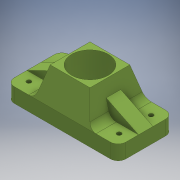
# Autodesk Inventor part: sujetador guia ejercedor presion
Saved by Autodesk Inventor 2018 (Build 220112000, 112)
## iProperties
Created: 2019-05-18
Part Number: sujetador guia ejercedor presion
Material: Generic
Document SubType Name: Modeling
Designer: JLVega003
Density: 1 g/cm^3
Appearance: Olive Green
Author: JLVega003
Autodesk Inventor part; units mm, degrees
ref_plane "YZ Plane" through (0, 0, 0) normal (1, 0, 0) x (0, 1, 0)
ref_plane "XZ Plane" through (0, 0, 0) normal (0, 1, 0) x (-1, 0, 0)
sketch "Sketch1" plane through (0, 0, 0) normal (0, 0, 1) x (1, 0, 0)
  line L0 (57.5, -28.5) -> (-57.5, -28.5)
  line L1 (-57.5, -28.5) -> (-57.5, 28.5)
  line L2 (-57.5, 28.5) -> (57.5, 28.5)
  line L3 (57.5, 28.5) -> (57.5, -28.5)
  line L4 (57.5, -28.5) -> (-57.5, 28.5) construction
  line L5 (-57.5, -28.5) -> (57.5, 28.5) construction
  line L6 (46.5, -16.5) -> (-46.5, -16.5) construction
  line L7 (-46.5, -16.5) -> (-46.5, 16.5) construction
  line L8 (-46.5, 16.5) -> (46.5, 16.5) construction
  line L9 (46.5, 16.5) -> (46.5, -16.5) construction
  line L10 (46.5, -16.5) -> (-46.5, 16.5) construction
  line L11 (-46.5, -16.5) -> (46.5, 16.5) construction
  line L12 (36, -11.5) -> (-36, -11.5) construction
  line L13 (-36, -11.5) -> (-36, 11.5) construction
  line L14 (-36, 11.5) -> (36, 11.5) construction
  line L15 (36, 11.5) -> (36, -11.5) construction
  line L16 (36, -11.5) -> (-36, 11.5) construction
  line L17 (-36, -11.5) -> (36, 11.5) construction
  circle A0 centre (-46.5, 16.5) radius 2.25
  circle A1 centre (-46.5, -16.5) radius 2.25
  circle A2 centre (46.5, -16.5) radius 2.25
  circle A3 centre (46.5, 16.5) radius 2.25
  point P0 (0, 0)
  dimension "d0" = 115
  dimension "d1" = 57
  dimension "d2" = 93
  dimension "d3" = 33
  dimension "d4" = 72
  dimension "d5" = 23
  dimension "d6" = 4.5
  constraints: 36 end point, 6 midpoint, 6 parallel, 4 centre point, 4 coincident, 3 equal radius, 3 horizontal, 3 perpendicular
  measures "d0" distance of L1.end L2.end
  measures "d1" distance of L0.end L1.end
  measures "d2" distance of L7.end L8.end
  measures "d3" distance of L6.end L7.end
  measures "d4" distance of L13.end L14.end
  measures "d5" distance of L12.end L13.end
  measures "d6" diameter of A0
extrude "Extrusion1" add sketch "Sketch1" along normal blind 15
sketch "Sketch6" plane through (0, 0, 15) normal (0, 0, 1) x (1, 0, 0)
  line L0 (57.5, 28.5) -> (-57.5, 28.5) projected
  line L1 (28.5, -28.5) -> (-28.5, -28.5)
  line L2 (-28.5, -28.5) -> (-28.5, 28.5)
  line L3 (-28.5, 28.5) -> (28.5, 28.5)
  line L4 (28.5, 28.5) -> (28.5, -28.5)
  line L5 (28.5, -28.5) -> (-28.5, 28.5) construction
  line L6 (-28.5, -28.5) -> (28.5, 28.5) construction
  point P0 (0, 0)
  dimension "d27" = 57
  constraints: 12 end point, 2 midpoint, 2 parallel, 1 horizontal, 1 perpendicular, 1 point on line
  measures "d27" distance of L2.end L3.end
ref_plane "Work Plane1" through (0, 0, 45) normal (0, 0, 1) x (1, 0, 0)
sketch "Sketch7" plane through (0, 0, 45) normal (0, 0, 1) x (1, 0, 0)
  line L0 (20.5, -20.5) -> (-20.5, -20.5)
  line L1 (-20.5, -20.5) -> (-20.5, 20.5)
  line L2 (-20.5, 20.5) -> (20.5, 20.5)
  line L3 (20.5, 20.5) -> (20.5, -20.5)
  line L4 (20.5, -20.5) -> (-20.5, 20.5) construction
  line L5 (-20.5, -20.5) -> (20.5, 20.5) construction
  point P0 (0, 0)
  dimension "d29" = 41
  dimension "d30" = 41
  constraints: 12 end point, 2 midpoint, 2 parallel, 1 horizontal, 1 perpendicular
  measures "d29" distance of L1.end L2.end
  measures "d30" distance of L0.end L1.end
loft "Loft1" add profiles "Sketch6", "Sketch7"
fillet "Fillet2" radius 8 2 edges at (28.5, 0, 15) (-28.5, 0, 15)
sketch "Sketch8" plane through (0, 0, 0) normal (0, 1, 0) x (-1, 0, 0)
  line L0 (-34.6462, 15) -> (34.6462, 15) projected
  arc A0 (26.9163, 20.9387) -> (34.6462, 15) centre (34.6462, 23) ccw projected
  line L1 (26.9163, 20.9387) -> (20.5, 45) projected
  line L2 (20.5, 45) -> (-20.5, 45) projected
  line L3 (-26.9163, 20.9387) -> (-20.5, 45) projected
  arc A1 (-34.6462, 15) -> (-26.9163, 20.9387) centre (-34.6462, 23) ccw projected
  line L4 (57.5, 0) -> (-57.5, 0) projected
  line L5 (57.5, 0) -> (57.5, 15) projected
  line L6 (34.6462, 15) -> (57.5, 15) projected
  line L7 (-34.6462, 15) -> (34.6462, 15) projected
  line L8 (-57.5, 15) -> (-34.6462, 15) projected
  line L9 (-57.5, 0) -> (-57.5, 15) projected
  line L10 (57.5, 15) -> (24.1643, 31.2589)
  line L11 (26.9163, 20.9387) -> (20.5, 45) projected
  line L12 (24.1643, 31.2589) -> (24.1643, 15)
  line L13 (57.5, 0) -> (57.5, 15) projected
  line L14 (24.1643, 15) -> (57.5, 15)
  line L15 (-57.5, 15) -> (-24.1643, 31.2589)
  line L16 (-24.1643, 31.2589) -> (-24.1643, 15)
  line L17 (-34.6462, 15) -> (34.6462, 15) projected
  line L18 (-57.5, 15) -> (-34.6462, 15) projected
  line L19 (-24.1643, 15) -> (-57.5, 15)
  point P0 (0, 0)
  dimension "d36" = 26
  dimension "d37" = 26
  constraints: 12 end point, 4 point on line, 2 perpendicular, 1 collinear, 1 horizontal
  measures "d36" angle of L14 L10
  measures "d37" angle of L15 L0
extrude "Extrusion5" add sketch "Sketch8" along normal mid plane 15 contours A1 L3 L16 L0 | L8 L15 L3 A1 | L16 L3 L2 L1 L12 L0 | A0 L1 L10 L6
fillet "Fillet3" radius 8 4 edges at (-57.5, 28.5, 7.5) (-57.5, -28.5, 7.5) (57.5, -28.5, 7.5) (57.5, 28.5, 7.5)
sketch "Sketch9" plane through (0, 0, 0) normal (0, 1, 0) x (-1, 0, 0)
  line L0 (0, -9) -> (0, 54) projected
  line L1 (0, 0) -> (0, 45)
  line L2 (20.5, 45) -> (-20.5, 45) projected
  line L3 (0, 45) -> (-18.9, 45)
  line L4 (-18.9, 45) -> (-18.9, 15)
  line L5 (-18.9, 15) -> (-20.5, 15)
  line L6 (-20.5, 15) -> (-20.5, 0)
  line L7 (-20.5, 0) -> (0, 0)
  dimension "d41" = 37.8
  dimension "d42" = 41
  dimension "d43" = 15
  constraints: 12 end point, 3 perpendicular, 1 midpoint, 1 point on line, 1 vertical
  measures "d41" diameter of L4 L0
  measures "d42" diameter of L6 L0
  measures "d43" distance between parallel lines of L7 L5
revolve "Revolution2" cut sketch "Sketch9" angle 360 about axis through (0, 0, -10) along (0, 0, 1)
equation "\"d37\" = d36"
body "Solid1"
